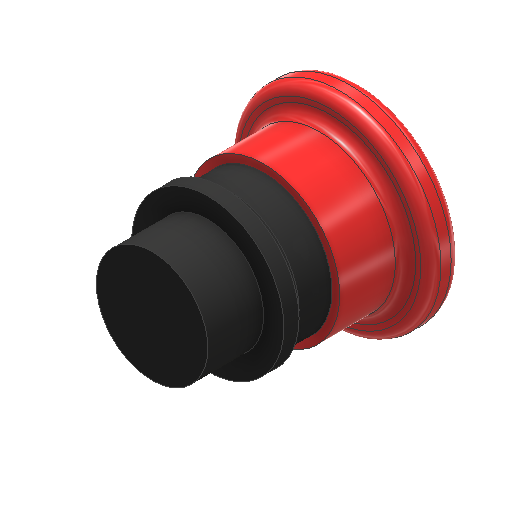
# Autodesk Inventor part: COTS_GENERIC_22mm_Safety_Switch
Saved by Autodesk Inventor 2026.1 (Build 301233000, 233)
## iProperties
Created: 2016-07-19
Part Number: COTS_GENERIC_22mm_Safety_Switch
Material: Ogólny
Document SubType Name: Modeling
Designer: Andrzej
Density: 1 g/cm^3
Appearance: Domyślna
Author: Andrzej
Autodesk Inventor part; units mm, degrees
ref_plane "YZ Plane" through (0, 0, 0) normal (1, 0, 0) x (0, 1, 0)
ref_plane "XZ Plane" through (0, 0, 0) normal (0, 1, 0) x (-1, 0, 0)
ref_plane "XY Plane" through (0, 0, 0) normal (0, 0, 1) x (1, 0, 0)
sketch "Szkic1" plane through (0, 0, 0) normal (0, 0, 1) x (1, 0, 0)
  line L0 (0, 5) -> (20, 5)
  line L1 (20, 5) -> (20, -1)
  line L2 (20, -1) -> (15, -1)
  line L3 (15, -1) -> (15, -14)
  line L4 (15, -14) -> (13.5, -14)
  line L5 (13.5, -14) -> (13.5, -22)
  line L6 (13.5, -22) -> (15, -22)
  line L7 (15, -22) -> (15, -25)
  line L8 (15, -25) -> (11, -25)
  line L9 (11, -25) -> (11, -36)
  line L10 (11, -36) -> (0, -36)
  line L11 (0, -36) -> (0, 5)
  line L12 (0, -44.2) -> (0, 13.2) projected
  point P0 (0, 0)
  dimension "d0" = 20
  dimension "d1" = 6
  dimension "d2" = 5
  dimension "d3" = 13
  dimension "d4" = 1.5
  dimension "d5" = 8
  dimension "d6" = 3
  dimension "d7" = 1.5
  dimension "d8" = 4
  dimension "d9" = 11
  constraints: 24 end point, 8 perpendicular, 2 horizontal, 1 parallel, 1 point on line, 1 vertical
  measures "d0" distance of L0.start L0.end
  measures "d1" distance of L0.end L1.end
  measures "d2" distance of L1.end L2.end
  measures "d3" distance of L2.end L3.end
  measures "d4" distance of L3.end L4.end
  measures "d5" distance of L4.end L5.end
  measures "d6" distance of L6.end L7.end
  measures "d7" distance of L5.end L6.end
  measures "d8" distance of L7.end L8.end
  measures "d9" distance of L8.end L9.end
revolve "Obrót1" add sketch "Szkic1" angle 360 about axis through (0, -10, 0) along (0, 1, 0)
chamfer "Faza1" distance 1.5 angle 45 1 edges at (-13.5, -22, 0)
fillet "Zaokrąglenie1" radius 2 3 edges at (-20, 5, 0) (-20, -1, 0) (-15, -1, 0)
